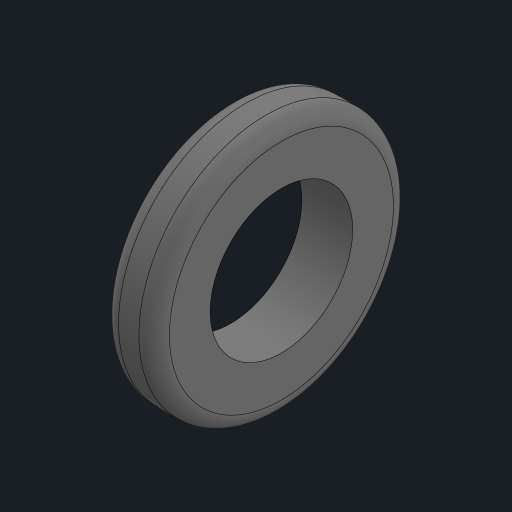
# Autodesk Inventor part: tire_o
Saved by Autodesk Inventor 2023 (Build 270158000, 158)
## iProperties
Created: 2022-06-17
Part Number: tire_o
Material: 一般
Document SubType Name: Modeling
Designer: legot
Density: 1 g/cm^3
Appearance: 既定
Author: legot
Autodesk Inventor part; units mm, degrees
ref_plane "YZ Plane" through (0, 0, 0) normal (1, 0, 0) x (0, 1, 0)
ref_plane "XZ Plane" through (0, 0, 0) normal (0, 1, 0) x (-1, 0, 0)
ref_plane "XY Plane" through (0, 0, 0) normal (0, 0, 1) x (1, 0, 0)
sketch "スケッチ1" plane through (0, 0, 0) normal (1, 0, 0) x (0, 1, 0)
  circle A0 centre (0, 0) radius 14
  circle A1 centre (0, 0) radius 25
  dimension "d0" = 28
  dimension "d1" = 50
  constraints: 2 centre point, 1 coincident
  measures "d0" diameter of A0
  measures "d1" diameter of A1
extrude "押し出し1" add sketch "スケッチ1" along normal mid plane 10
fillet "フィレット1" radius 3 2 edges at (5, -25, 0) (-5, -25, 0)
